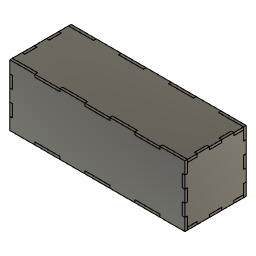
box (Autodesk Fusion 360 design; units mm, degrees)
Autodesk Fusion 360 part; units mm, degrees
note: some values were not read from the file. Set by a fixed rule: which sketch regions a step uses.
sketch "Sketch1" plane through (0, 0, 0) normal (0, 1, 0) x (1, 0, 0) in component "Front"
  line L0 (0, 0) -> (200, 0)
  line L1 (200, 0) -> (200, -70)
  line L2 (200, -70) -> (0, -70)
  line L3 (0, -70) -> (0, 0)
  line L4 (0, -6) -> (200, -6) construction
  line L5 (0, -3) -> (200, -3) construction
  line L6 (3, -70) -> (3, 0) construction
  line L7 (6, -50) -> (6, 0) construction
  line L8 (0, -56) -> (3, -56)
  line L9 (3, -56) -> (3, -42)
  line L10 (3, -42) -> (0, -42)
  line L11 (0, -42) -> (0, -56)
  line L12 (0, -28) -> (3, -28)
  line L13 (3, -28) -> (3, -14)
  line L14 (3, -14) -> (0, -14)
  line L15 (0, -14) -> (0, -28)
  line L16 (28.5714, -3) -> (57.1429, -3)
  line L17 (57.1429, -3) -> (57.1429, 0)
  line L18 (57.1429, 0) -> (28.5714, 0)
  line L19 (28.5714, 0) -> (28.5714, -3)
  line L20 (85.7143, -3) -> (114.2857, -3)
  line L21 (114.2857, -3) -> (114.2857, 0)
  line L22 (114.2857, 0) -> (85.7143, 0)
  line L23 (85.7143, 0) -> (85.7143, -3)
  line L24 (142.8571, -3) -> (171.4286, -3)
  line L25 (171.4286, -3) -> (171.4286, 0)
  line L26 (171.4286, 0) -> (142.8571, 0)
  line L27 (142.8571, 0) -> (142.8571, -3)
  line L28 (100, -70) -> (100, 0) construction
  line L29 (194, -50) -> (194, 0) construction
  line L30 (200, -56) -> (197, -56)
  line L31 (197, -56) -> (197, -42)
  line L32 (197, -42) -> (200, -42)
  line L33 (200, -28) -> (197, -28)
  line L34 (197, -14) -> (200, -14)
  line L35 (197, -28) -> (197, -14)
  line L36 (197, -70) -> (197, 0) construction
  dimension "d70" = 200
  dimension "d71" = 70
  dimension "d72" = 3
  dimension "d73" = 3
  dimension "d74" = 3
  dimension "d76" = 3
  dimension "d77" = 28.5714
  dimension "d78" = 28.5714
  dimension "d79" = 28.5714
  dimension "d80" = 28.5714
  dimension "d81" = 28.5714
  dimension "d82" = 28.5714
  dimension "d83" = 14
  dimension "d84" = 14
  dimension "d85" = 14
  dimension "d86" = 14
  constraint horizontal L0
  constraint vertical L1
  constraint horizontal L2
  constraint vertical L3
  constraint coincident L0.start L3.end
  constraint coincident L3 L4.start
  constraint coincident L1 L4.end
  constraint perpendicular L1 L4
  constraint coincident L3 L5.start
  constraint coincident L1 L5.end
  constraint perpendicular L1 L5
  constraint coincident L2 L6.start
  constraint coincident L0 L6.end
  constraint perpendicular L0 L6
  constraint coincident L0 L7.end
  constraint perpendicular L0 L7
  constraint horizontal L8
  constraint vertical L9
  constraint horizontal L10
  constraint vertical L11
  constraint coincident L6 L9.end
  constraint coincident L3 L8.start
  constraint horizontal L12
  constraint vertical L13
  constraint horizontal L14
  constraint vertical L15
  constraint coincident L6 L13.end
  constraint coincident L3 L12.start
  constraint horizontal L16
  constraint vertical L17
  constraint horizontal L18
  constraint vertical L19
  constraint coincident L0 L17.end
  constraint coincident L5 L16.start
  constraint horizontal L20
  constraint vertical L21
  constraint horizontal L22
  constraint vertical L23
  constraint coincident L0 L21.end
  constraint coincident L5 L20.start
  constraint horizontal L24
  constraint vertical L25
  constraint horizontal L26
  constraint vertical L27
  constraint coincident L0 L25.end
  constraint coincident L5 L24.start
  constraint midpoint L2 L28.start
  constraint midpoint L0 L28.end
  constraint symmetric L6.start L28 L36.start
  constraint symmetric L6.end L28 L36.end
  constraint symmetric L7.start L28 L29.start
  constraint symmetric L7.end L28 L29.end
  constraint symmetric L8.start L28 L30.start
  constraint symmetric L8.end L28 L30.end
  constraint symmetric L9.end L28 L31.end
  constraint symmetric L10.end L28 L32.end
  constraint symmetric L12.start L28 L33.start
  constraint symmetric L12.end L28 L33.end
  constraint symmetric L13.end L28 L34.start
  constraint symmetric L14.end L28 L34.end
  measures "d70" distance of L0.start L0.end
  measures "d71" distance of L0.start L2.end
  measures "d72" distance of L0 L5
  measures "d73" distance of L4 L5
  measures "d74" distance of L3 L6
  measures "d76" distance of L6 L7
  measures "d77" distance of L3 L19
  measures "d78" distance of L17 L19
  measures "d79" distance of L17 L23
  measures "d80" distance of L21 L23
  measures "d81" distance of L21 L27
  measures "d82" distance of L25 L27
  measures "d83" distance of L0 L14
  measures "d84" distance of L12 L14
  measures "d85" distance of L10 L12
  measures "d86" distance of L8 L10
extrude "Extrude1" add sketch "Sketch1" along normal blind 3 contours L0 L1 L2 L3 L8 L9 L10 L12 L13 L14 L16 L17 L19 L20 L21 L23 L24 L25 L27 L30 L31 L32 L33 L34 L35 makes body 1 in component "Front"
sketch "Sketch4" plane through (0, 0, 0) normal (-1, 0, 0) x (0, -1, 0) in component "Left"
  line L0 (0, 0) -> (0, 14)
  line L1 (0, 14) -> (-3, 14)
  line L2 (-3, 14) -> (-3, 0)
  line L3 (-3, 0) -> (0, 0)
  line L4 (0, 0) -> (-70, 0)
  line L5 (-70, 0) -> (-70, 70)
  line L6 (-70, 70) -> (0, 70)
  line L7 (0, 70) -> (0, 0)
  line L8 (-3, 70) -> (-3, 0) construction
  line L9 (-6, 70) -> (-6, 0) construction
  line L10 (0, 3) -> (-70, 3) construction
  line L11 (0, 14) -> (-1.5, 14) construction
  line L12 (0, 6) -> (-70, 6) construction
  line L13 (-3, 14) -> (0, 14)
  line L14 (0, 14) -> (0, 0)
  line L15 (0, 0) -> (-3, 0)
  line L16 (-3, 0) -> (-3, 14)
  line L17 (-3, 42) -> (0, 42)
  line L18 (0, 42) -> (0, 28)
  line L19 (0, 28) -> (-3, 28)
  line L20 (-3, 28) -> (-3, 42)
  line L21 (-3, 70) -> (0, 70)
  line L22 (0, 70) -> (0, 56)
  line L23 (0, 56) -> (-3, 56)
  line L24 (-3, 56) -> (-3, 70)
  line L25 (0, 0) -> (-14, 0)
  line L26 (-14, 0) -> (-14, 3)
  line L27 (-14, 3) -> (0, 3)
  line L28 (0, 3) -> (0, 0)
  line L29 (-28, 3) -> (-42, 3)
  line L30 (-42, 3) -> (-42, 0)
  line L31 (-42, 0) -> (-28, 0)
  line L32 (-28, 0) -> (-28, 3)
  line L33 (-70, 0) -> (-56, 0)
  line L34 (-56, 0) -> (-56, 3)
  line L35 (-56, 3) -> (-70, 3)
  line L36 (-70, 3) -> (-70, 0)
  line L37 (-35, 70) -> (-35, 0) construction
  line L38 (-64, 70) -> (-64, 0) construction
  line L39 (-70, 28) -> (-67, 28)
  line L40 (-67, 42) -> (-70, 42)
  line L41 (-70, 56) -> (-67, 56)
  line L42 (-67, 70) -> (-70, 70)
  line L43 (-67, 56) -> (-67, 70)
  line L44 (-67, 28) -> (-67, 42)
  line L45 (-67, 0) -> (-67, 14)
  line L46 (-67, 70) -> (-67, 0) construction
  line L47 (-67, 14) -> (-70, 14)
  line L48 (-70, 0) -> (-67, 0)
  dimension "d91" = 70
  dimension "d92" = 70
  dimension "d95" = 3
  dimension "d96" = 3
  dimension "d97" = 3
  dimension "d98" = 3
  dimension "d99" = 14
  dimension "d100" = 14
  dimension "d101" = 14
  dimension "d103" = 14
  dimension "d104" = 14
  dimension "d105" = 14
  dimension "d106" = 14
  dimension "d107" = 14
  constraint horizontal L4
  constraint vertical L5
  constraint horizontal L6
  constraint vertical L7
  constraint coincident L0.start L3.end
  constraint coincident L6 L8.start
  constraint coincident L4 L2.end
  constraint perpendicular L4 L8
  constraint coincident L6 L9.start
  constraint coincident L4 L9.end
  constraint perpendicular L4 L9
  constraint coincident L7 L10.start
  constraint coincident L5 L10.end
  constraint perpendicular L5 L10
  constraint coincident L0.end L1.start
  constraint midpoint L1 L11.end
  constraint coincident L7 L12.start
  constraint coincident L5 L12.end
  constraint perpendicular L5 L12
  constraint horizontal L13
  constraint vertical L14
  constraint horizontal L15
  constraint vertical L16
  constraint coincident L8 L1.end
  constraint horizontal L17
  constraint vertical L18
  constraint horizontal L19
  constraint vertical L20
  constraint coincident L7 L18.end
  constraint coincident L8 L17.start
  constraint horizontal L21
  constraint vertical L22
  constraint horizontal L23
  constraint vertical L24
  constraint coincident L7 L22.end
  constraint horizontal L25
  constraint vertical L26
  constraint horizontal L27
  constraint vertical L28
  constraint coincident L10 L26.end
  constraint horizontal L29
  constraint vertical L30
  constraint horizontal L31
  constraint vertical L32
  constraint coincident L4 L30.end
  constraint coincident L10 L29.start
  constraint horizontal L33
  constraint vertical L34
  constraint horizontal L35
  constraint vertical L36
  constraint coincident L10 L34.end
  constraint midpoint L6 L37.start
  constraint midpoint L31 L37.end
  constraint symmetric L0.start L37 L4.end
  constraint symmetric L8.start L37 L42.start
  constraint symmetric L2.end L37 L45.start
  constraint symmetric L9.start L37 L38.start
  constraint symmetric L9.end L37 L38.end
  constraint symmetric L1.end L37 L45.end
  constraint symmetric L0.end L37 L47.end
  constraint symmetric L17.start L37 L40.start
  constraint symmetric L17.end L37 L40.end
  constraint symmetric L18.end L37 L39.start
  constraint symmetric L19.end L37 L39.end
  constraint symmetric L6.end L37 L5.end
  constraint symmetric L22.end L37 L41.start
  constraint symmetric L23.end L37 L41.end
  measures "d91" distance of L0.start L4.end
  measures "d92" distance of L0.start L6.end
  measures "d95" distance of L7 L8
  measures "d96" distance of L8 L9
  measures "d97" distance of L4 L10
  measures "d98" distance of L10 L12
  measures "d99" distance of L4 L13
  measures "d100" distance of L13 L19
  measures "d101" distance of L17 L19
  measures "d103" distance of L6 L23
  measures "d104" distance of L26 L28
  measures "d105" distance of L26 L32
  measures "d106" distance of L30 L32
  measures "d107" distance of L30 L34
extrude "Extrude1'" add sketch "Sketch4" against normal blind 3 separate body contours L1 L2 L4 L5 L6 L7 L13 L16 L17 L19 L20 L23 L24 L26 L27 L29 L30 L32 L34 L35 L39 L40 L41 L43 L44 L45 L47 makes body 2 in component "Left"
ref_plane "WorkPlane1" through (100, 1.5, 7) normal (-1, 0, 0) x (0, 0, 1)
mirror "MirrorComponent1" about plane through (0, 0, 0) normal (0, 0, 1) of bodies 2 makes body 3 in component "Right"
ref_plane "WorkPlane2" through (1.5, 35, 21) normal (0, -1, 0) x (0, 0, -1)
mirror "MirrorComponent2" about plane through (0, 0, 0) normal (0, 0, 1) of bodies 1 makes body 4 in component "Back"
mirror "MirrorComponent2'" about plane through (0, 0, 0) normal (0, 0, 1) of bodies 2 makes body 5 in component "Left(Mirror) (1)"
sketch "Sketch1 (2)" plane through (0, 0, 3) normal (0, 0, -1) x (1, 0, 0) in component "Base"
  line L0 (0, 0) -> (200, 0)
  line L1 (200, 0) -> (200, -70)
  line L2 (200, -70) -> (0, -70)
  line L3 (0, -70) -> (0, 0)
  dimension "d110" = 70
  dimension "d111" = 200
  constraint horizontal L0
  constraint vertical L1
  constraint horizontal L2
  constraint vertical L3
  constraint coincident L0.start L3.end
  measures "d110" distance of L0.start L2.end
  measures "d111" distance of L1 L3
extrude "Extrude1''" add sketch "Sketch1 (2)" along normal blind 3 separate body makes body 6 in component "Base"
combine "Combine1" operation cut target body 6 tool bodies 4 2 1 3 body 4 seen with x (1, 0, 0) y (0, -1, 0) z (0, 0, -1) at (0, 70, 0) body 3 seen with x (-1, 0, 0) y (0, 1, 0) z (0, 0, -1) at (200, 0, 0) keep tools in component "Base"
ref_plane "WorkPlane4" through (100, 35, 35) normal (0, 0, -1) x (-1, 0, 0)
mirror "MirrorComponent3" about plane through (0, 0, 0) normal (0, 0, 1) of bodies 6 makes body 7 in component "Base(Mirror)"
mirror "MirrorComponent4" about plane through (0, 0, 0) normal (0, 0, 1) of bodies 6 makes body 8 in component "Top"
combine "Combine1'" operation cut target body 3 tool bodies 8 body 8 seen with x (-1, 0, 0) y (0, 1, 0) z (0, 0, -1) at (200, 0, -70) keep tools in component "Right"
combine "Combine1''" operation cut target body 1 tool bodies 8 body 8 seen with x (1, 0, 0) y (0, 1, 0) z (0, 0, 1) at (0, 0, 70) keep tools in component "Front"
combine "Combine1'''" operation cut target body 2 tool bodies 8 body 8 seen with x (1, 0, 0) y (0, 1, 0) z (0, 0, 1) at (0, 0, 70) keep tools in component "Left"
combine "Combine1''''" operation cut target body 4 tool bodies 8 body 8 seen with x (1, 0, 0) y (0, -1, 0) z (0, 0, -1) at (0, 70, -70) keep tools in component "Back"
sketch "Sketch1 (3)" plane through (0, 0, 0) normal (0, 0, 1) x (-1, 0, 0) in component "Top"
  line L0 (-197, -56) -> (-200, -56)
  line L1 (-200, -56) -> (-200, -67)
  line L2 (-200, -67) -> (-171.4286, -67)
  line L3 (-171.4286, -67) -> (-171.4286, -70)
  line L4 (-171.4286, -70) -> (-142.8571, -70)
  line L5 (-142.8571, -70) -> (-142.8571, -67)
  line L6 (-142.8571, -67) -> (-114.2857, -67)
  line L7 (-114.2857, -67) -> (-114.2857, -70)
  line L8 (-114.2857, -70) -> (-85.7143, -70)
  line L9 (-85.7143, -70) -> (-85.7143, -67)
  line L10 (-85.7143, -67) -> (-57.1429, -67)
  line L11 (-57.1429, -67) -> (-57.1429, -70)
  line L12 (-57.1429, -70) -> (-28.5714, -70)
  line L13 (-28.5714, -70) -> (-28.5714, -67)
  line L14 (-28.5714, -67) -> (0, -67)
  line L15 (0, -67) -> (0, -56)
  line L16 (0, -56) -> (-3, -56)
  line L17 (-3, -56) -> (-3, -42)
  line L18 (-3, -42) -> (0, -42)
  line L19 (0, -42) -> (0, -28)
  line L20 (0, -28) -> (-3, -28)
  line L21 (-3, -28) -> (-3, -14)
  line L22 (-3, -14) -> (0, -14)
  line L23 (0, -14) -> (0, -3)
  line L24 (0, -3) -> (-28.5714, -3)
  line L25 (-28.5714, -3) -> (-28.5714, 0)
  line L26 (-28.5714, 0) -> (-57.1429, 0)
  line L27 (-57.1429, 0) -> (-57.1429, -3)
  line L28 (-57.1429, -3) -> (-85.7143, -3)
  line L29 (-85.7143, -3) -> (-85.7143, 0)
  line L30 (-85.7143, 0) -> (-114.2857, 0)
  line L31 (-114.2857, 0) -> (-114.2857, -3)
  line L32 (-114.2857, -3) -> (-142.8571, -3)
  line L33 (-142.8571, -3) -> (-142.8571, 0)
  line L34 (-142.8571, 0) -> (-171.4286, 0)
  line L35 (-171.4286, 0) -> (-171.4286, -3)
  line L36 (-171.4286, -3) -> (-200, -3)
  line L37 (-200, -3) -> (-200, -14)
  line L38 (-200, -14) -> (-197, -14)
  line L39 (-197, -14) -> (-197, -28)
  line L40 (-197, -28) -> (-200, -28)
  line L41 (-200, -28) -> (-200, -42)
  line L42 (-200, -42) -> (-197, -42)
  line L43 (-197, -42) -> (-197, -56)
  line L44 (0, 0) -> (-200, 0)
  line L45 (-200, 0) -> (-200, -70)
  line L46 (-200, -70) -> (0, -70)
  line L47 (0, -70) -> (0, 0)
  line L48 (-100, -70) -> (-100, 0)
  line L49 (0, -35) -> (-150, -35)
  line L50 (-60, -33.5) -> (-90, -33.5)
  line L51 (-90, -33.5) -> (-90, -36.5)
  line L52 (-90, -36.5) -> (-60, -36.5)
  line L53 (-60, -36.5) -> (-60, -33.5)
  line L54 (-60, -33.5) -> (-90, -36.5) construction
  line L55 (-90, -33.5) -> (-60, -36.5) construction
  point P0 (-75, -35)
  dimension "d118" = 200
  dimension "d119" = 70
  dimension "d124" = 30
  dimension "d125" = 3
  constraint horizontal L44
  constraint vertical L45
  constraint horizontal L46
  constraint vertical L47
  constraint coincident L44.start L47.end
  constraint vertical L48
  constraint midpoint L8 L48.start
  constraint horizontal L49
  constraint midpoint L47 L49.start
  constraint horizontal L50
  constraint perpendicular L50 L51
  constraint parallel L50 L52
  constraint parallel L51 L53
  constraint coincident L54 P0
  constraint coincident L55 P0
  constraint midpoint L49 P0
  measures "d118" distance of L44.start L44.end
  measures "d119" distance of L44.start L46.end
  measures "d124" distance of L51.end L52.end
  measures "d125" distance of L50.end L51.end
component "Front" placed x (1, 0, 0) y (0, 1, 0) z (0, 0, 1) at (0, 0, 0)
component "Left" placed x (1, 0, 0) y (0, 1, 0) z (0, 0, 1) at (0, 0, 0)
component "Base" placed x (1, 0, 0) y (0, 1, 0) z (0, 0, 1) at (0, 0, 0)
component "Right" placed x (-1, 0, 0) y (0, 1, 0) z (0, 0, -1) at (200, 0, 0)
component "Back" placed x (1, 0, 0) y (0, -1, 0) z (0, 0, -1) at (0, 70, 0)
component "Top" placed x (1, 0, 0) y (0, 1, 0) z (0, 0, 1) at (0, 0, 70)
equation "length = 200 mm" comment "Box Length"
equation "width = 70 mm" comment "Box Width"
equation "height = 70 mm" comment "Box Height"
equation "thickness = 3 mm" comment "Box Thickness"
equation "nthw = 5" comment "No. of tabs(h/w)"
equation "ntl = 7" comment "No. of tabs(l)"
equation "d70 = length"
equation "d71 = height"
equation "d72 = thickness"
equation "d73 = thickness"
equation "d74 = thickness"
equation "d76 = thickness"
equation "d77 = length / ntl"
equation "d78 = d77"
equation "d79 = d78"
equation "d80 = d79"
equation "d81 = d80"
equation "d82 = d81"
equation "d83 = height / nthw"
equation "d84 = d83"
equation "d85 = d84"
equation "d86 = d85"
equation "d87 = thickness"
equation "d91 = width"
equation "d92 = height"
equation "d95 = thickness"
equation "d96 = thickness"
equation "d97 = thickness"
equation "d98 = thickness"
equation "d99 = height / nthw"
equation "d100 = d99"
equation "d101 = d100"
equation "d103 = d101"
equation "d104 = width / nthw"
equation "d105 = d104"
equation "d106 = d105"
equation "d107 = d106"
equation "d108 = -thickness"
equation "d110 = width"
equation "d111 = length"
equation "d112 = thickness"
equation "d118 = length"
equation "d119 = width"
equation "slength = 30 mm" comment "Length of Slot"
equation "swidth = 3 mm" comment "Width of Slot"
equation "d124 = slength"
equation "d125 = swidth"
